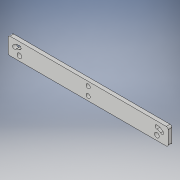
# Autodesk Inventor part: CameraBase
Saved by Autodesk Inventor 2019 (Build 230136000, 136)
## iProperties
Created: 2019-07-15
Part Number: CameraBase
Material: Generic
Document SubType Name: Modeling
Designer: aorfi
Density: 1 g/cm^3
Appearance: Default
Author: aorfi
Autodesk Inventor part; units mm, degrees
ref_plane "YZ Plane" through (0, 0, 0) normal (1, 0, 0) x (0, 1, 0)
ref_plane "XZ Plane" through (0, 0, 0) normal (0, 1, 0) x (-1, 0, 0)
ref_plane "XY Plane" through (0, 0, 0) normal (0, 0, 1) x (1, 0, 0)
sketch "Sketch1" plane through (0, 0, 0) normal (0, 0, 1) x (1, 0, 0)
  line L0 (-85, -9) -> (85, -9)
  line L1 (85, -9) -> (85, 9)
  line L2 (85, 9) -> (-85, 9)
  line L3 (-85, 9) -> (-85, -9)
  line L4 (-85, -9) -> (85, 9) construction
  line L5 (85, -9) -> (-85, 9) construction
  point P0 (0, 0)
  dimension "d3" = 18
  dimension "d26" = 170
  constraints: 12 end point, 2 midpoint, 2 parallel, 1 horizontal, 1 perpendicular
  measures "d3" distance of L2.end L0.start
  measures "d26" distance of L0.start L0.end
extrude "Extrusion1" add sketch "Sketch1" along normal mid plane 4
sketch "Sketch2" plane through (0, 0, -2) normal (0, 0, -1) x (-1, 0, 0)
  line L0 (0, -15) -> (0, 15) construction
  line L1 (85, 9) -> (-85, 9) projected
  circle A0 centre (73, -4) radius 2.5
  arc A1 (73, 5.3986) -> (73, 1.6013) centre (73, 3.5) ccw
  line L2 (73, 3.5) -> (73, -4) construction
  line L3 (73, -4) -> (78.3033, -4) construction
  circle A2 centre (73, -4) radius 7.5 construction
  arc A3 (76.9608, -0.0392) -> (79.6458, 2.6458) centre (78.3033, 1.3033) ccw
  arc A4 (79.6458, 2.6458) -> (73, 5.3986) centre (73, -4) ccw
  arc A5 (76.9608, -0.0392) -> (73, 1.6013) centre (73, -4) ccw
  line L4 (85, -10.7625) -> (85, 10.7625) construction
  line L5 (73, -4) -> (78.3033, 1.3033) construction
  line L6 (78.3033, 1.3033) -> (78.3033, -4) construction
  line L7 (85, -9) -> (85, 9) projected
  line L8 (-85, -9) -> (85, -9) projected
  line L9 (-73, 3.5) -> (-73, -4) construction
  arc A6 (-73, 1.6013) -> (-73, 5.3986) centre (-73, 3.5) ccw
  circle A7 centre (-73, -4) radius 2.5
  arc A8 (-73, 1.6013) -> (-76.9608, -0.0392) centre (-73, -4) ccw
  line L10 (-73, -4) -> (-78.3033, -4) construction
  line L11 (-73, -4) -> (-78.3033, 1.3033) construction
  line L12 (-78.3033, 1.3033) -> (-78.3033, -4) construction
  circle A9 centre (-73, -4) radius 7.5 construction
  arc A10 (-73, 5.3986) -> (-79.6458, 2.6458) centre (-73, -4) ccw
  arc A11 (-79.6458, 2.6458) -> (-76.9608, -0.0392) centre (-78.3033, 1.3033) ccw
  line L13 (-85, -10.7625) -> (-85, 10.7625) construction
  line L14 (-85, -9) -> (-85, 9)
  point P0 (0, 0)
  point P1 (85, 0)
  point P2 (-85, 0)
  dimension "d40" = 5
  dimension "d41" = 3.7973
  dimension "d42" = 3.7973
  dimension "d43" = 15
  dimension "d44" = 12
  dimension "d45" = 5
  constraints: 24 end point, 20 point on circle, 15 symmetric about line, 12 centre point, 8 coincident, 2 point on line, 2 tangent, 2 vertical, 1 collinear, 1 horizontal, 1 midpoint, 1 perpendicular, 1 vertical alignment, 6 other
  measures "d40" diameter of A0
  measures "d41" diameter of A1
  measures "d42" diameter of A3
  measures "d43" diameter of A2
  measures "d44" distance from line of L2.end L4
  measures "d45" distance between parallel lines of L8 L3
extrude "Extrusion2" cut sketch "Sketch2" against normal through all contours A0 | A4 A3 A5 A1 | A8 A11 A10 A6 | A7
fillet "Fillet1" radius 2 4 edges at (-85, 9, 0) (-85, -9, 0) (85, 9, 0) (85, -9, 0)
sketch "Sketch5" plane through (0, 0, 2) normal (0, 0, 1) x (1, 0, 0)
  line L0 (0, -9) -> (0, 0) construction
  line L1 (0, 0) -> (0, 9) construction
  line L2 (83, 9) -> (-83, 9) construction
  line L3 (-83, -9) -> (83, -9) construction
  point P0 (0, -4.5)
  point P1 (0, 4.5)
  constraints: 4 end point, 4 midpoint, 1 vertical
hole "Hole2" at (0, -4.5, 2) at (0, 4.5, 2) direction (0, 0, -1) diameter 4.496 end through all clearance for "Flat Head Machine Screw (82)" size "#8" standard "Ansi Unified Screw Threads"
equation "\"d42\" = d41"
body "Solid1"
